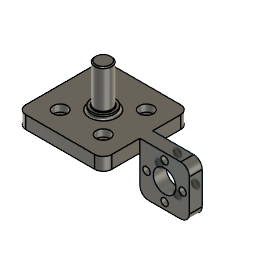
MGN12H_Carriage_Adapter (Autodesk Fusion 360 design; units mm, degrees)
part number: 2026-08-12-12-25-13-013
Autodesk Fusion 360 part; units mm, degrees
sketch "草图1" plane through (0, 0, 0) normal (0, 0, 1) x (1, 0, 0)
  line L0 (20, 20) -> (-20, 20)
  line L1 (-20, 20) -> (-20, -20)
  line L2 (-20, -20) -> (20, -20)
  line L3 (20, -20) -> (20, 20)
  line L4 (20, 20) -> (-20, -20) construction
  line L5 (-20, 20) -> (20, -20) construction
  dimension "d25" = 40
  dimension "d26" = 40
  constraint horizontal L0
  constraint perpendicular L0 L1
  constraint parallel L0 L2
  constraint parallel L1 L3
  constraint coincident L4 origin
  constraint coincident L5 origin
  measures "d25" distance of L0.start L0.end
  measures "d26" distance of L0.start L2.end
extrude "拉伸1" add sketch "草图1" along normal blind 6
fillet "圆角1" radius 4 4 edges at (-20, -20, 3) (20, -20, 3) (20, 20, 3) (-20, 20, 3)
sketch "草图2" plane through (0, 0, 6) normal (0, 0, 1) x (-1, 0, 0)
  arc A0 (16, -20) -> (20, -16) centre (16, -16) ccw
  line L0 (20, -16) -> (20, 16)
  arc A1 (20, 16) -> (16, 20) centre (16, 16) ccw
  line L1 (16, 20) -> (-16, 20)
  arc A2 (-16, 20) -> (-20, 16) centre (-16, 16) ccw
  line L2 (-20, 16) -> (-20, -16)
  arc A3 (-20, -16) -> (-16, -20) centre (-16, -16) ccw
  line L3 (-16, -20) -> (16, -20)
  point P0 (-10, -10)
  dimension "d31" = 10
  dimension "d32" = 10
  measures "d31" distance of L2 P0
  measures "d32" distance of L3 P0
hole "孔1" at (10, 10, 6) direction (0, 0, -1) diameter 3.4 depth 15 tip angle 118 counterbore diameter 6.5 counterbore depth 3.3
pattern_linear "R-阵列1" count 2 spacing 20 along (-1, 0, 0) count 2 spacing 20 along (0, -1, 0) of "孔1"
sketch "草图3" plane through (0, 0, 6) normal (0, 0, 1) x (-1, 0, 0)
  circle A0 centre (10, 10) radius 3.25
  circle A1 centre (-10, 10) radius 3.25
  circle A2 centre (10, -10) radius 3.25
  circle A3 centre (-10, -10) radius 3.25
  arc A4 (16, -20) -> (20, -16) centre (16, -16) ccw
  line L0 (20, -16) -> (20, 16)
  arc A5 (20, 16) -> (16, 20) centre (16, 16) ccw
  line L1 (16, 20) -> (-16, 20)
  arc A6 (-16, 20) -> (-20, 16) centre (-16, 16) ccw
  line L2 (-20, 16) -> (-20, -16)
  arc A7 (-20, -16) -> (-16, -20) centre (-16, -16) ccw
  line L3 (-16, -20) -> (16, -20)
  circle A8 centre (0, 0) radius 5.4
  dimension "d42" = 10.8
  constraint coincident A8.centre origin
  measures "d42" diameter of A8
extrude "拉伸2" add sketch "草图3" along normal blind 1.8 contours A8
fillet "圆角2" radius 1 1 edges at (5.0346, -1.9527, 6)
sketch "草图4" plane through (0, 0, 7.8) normal (0, 0, 1) x (-1, 0, 0)
  circle A0 centre (0, 0) radius 5.4
  circle A1 centre (0, 0) radius 3.95
  dimension "d47" = 7.9
  constraint coincident A0.centre A1.centre
  measures "d47" diameter of A1
extrude "拉伸3" add sketch "草图4" along normal blind 18 contours A1
fillet "圆角3" radius 0.3 1 edges at (3.6827, -1.4284, 7.8)
chamfer "倒角1" distance 0.5 angle 45 1 edges at (3.6827, 1.4284, 25.8)
sketch "草图5" plane through (0, 0, 0) normal (0, 1, 0) x (1, 0, 0)
sketch "草图6" plane through (0, 0, 0) normal (0, 0, 1) x (1, 0, 0)
  line L0 (20, -3) -> (43, -3)
  line L1 (43, -3) -> (43, 3)
  line L2 (43, 3) -> (20, 3)
  line L3 (20, 3) -> (20, -3)
  constraint horizontal L0
  constraint vertical L1
  constraint horizontal L2
  constraint vertical L3
extrude "拉伸4" add sketch "草图6" along normal blind 6 and the other way blind 17
sketch "草图7" plane through (0, 3, 0) normal (0, 1, 0) x (-1, 0, 0)
  line L0 (-20, 0) -> (-20, 6)
  line L1 (-20, 6) -> (-43, 6)
  line L2 (-43, 6) -> (-43, -17)
  line L3 (-43, -17) -> (-20, -17)
  line L4 (-20, -17) -> (-20, 0)
  circle A0 centre (-31.5, -5.5) radius 5.25
  line L5 (0, 20) -> (0, 2.5)
  dimension "d57" = 10.5
  dimension "d58" = 31.5
  dimension "d59" = 11.5
  measures "d57" diameter of A0
  measures "d58" distance of A0.centre L5
  measures "d59" distance of L1 A0.centre
extrude "拉伸5" cut sketch "草图7" against normal blind 6 contours A0
sketch "草图8" plane through (0, 3, 0) normal (0, 1, 0) x (-1, 0, 0)
  circle A0 centre (-31.5, -5.5) radius 5.25
  line L0 (-20, 0) -> (-20, 6)
  line L1 (-20, 6) -> (-43, 6)
  line L2 (-43, 6) -> (-43, -17)
  line L3 (-43, -17) -> (-20, -17)
  line L4 (-20, -17) -> (-20, 0)
  circle A1 centre (-31.5, 2.875) radius 1.7
  circle A2 centre (-31.5, -13.875) radius 1.7
  circle A3 centre (-39.875, -5.5) radius 1.7
  circle A4 centre (-23.125, -5.5) radius 1.7
  dimension "d62" = 3.4
  dimension "d64" = 3.125
  dimension "d67" = 11.5
  dimension "d68" = 3.4
  dimension "d69" = 3.125
  dimension "d70" = 11.5
  dimension "d71" = 3.4
  dimension "d72" = 3.4
  dimension "d73" = 3.125
  dimension "d74" = 3.125
  dimension "d75" = 11.5
  dimension "d76" = 11.5
  measures "d62" diameter of A1
  measures "d64" distance of L1 A1.centre
  measures "d67" distance of L0 A1.centre
  measures "d68" diameter of A2
  measures "d69" distance of L3 A2.centre
  measures "d70" distance of L4 A2.centre
  measures "d71" diameter of A3
  measures "d72" diameter of A4
  measures "d73" distance of L2 A3.centre
  measures "d74" distance of L4 A4.centre
  measures "d75" distance of L3 A3.centre
  measures "d76" distance of L3 A4.centre
extrude "拉伸7" cut sketch "草图8" against normal blind 6 contours A1 | A2 | A3 | A4
fillet "圆角4" radius 4 3 edges at (43, 0, 6) (43, 0, -17) (20, 0, -17)
equation "Base_Length = 40 mm" comment "Base length"
equation "Base_Width = 40 mm" comment "Base width"
equation "Base_Thickness = 6 mm" comment "Base thickness"
equation "Base_Corner_Radius = 4 mm" comment "Base corner radius"
equation "Hole_Pitch_X = 20 mm" comment "M3 hole pitch X"
equation "Hole_Pitch_Y = 20 mm" comment "M3 hole pitch Y"
equation "M3_Clearance_Diameter = 3.4 mm" comment "M3 clearance hole diameter"
equation "Counterbore_Diameter = 6.5 mm" comment "M3 socket-head counterbore diameter"
equation "Counterbore_Depth = 3.3 mm" comment "M3 counterbore depth"
equation "Shaft_Diameter = 7.9 mm" comment "Vertical printed shaft diameter"
equation "Shoulder_Diameter = 10.8 mm" comment "Bearing inner-ring support shoulder diameter"
equation "Shoulder_Height = 1.8 mm" comment "Bearing shoulder height"
equation "Shaft_Height = 18 mm" comment "Shaft height above shoulder"
equation "Shoulder_Base_Fillet = 1 mm" comment "Fillet between shoulder and base"
equation "Shaft_Shoulder_Fillet = 0.3 mm" comment "Small fillet between shaft and shoulder"
equation "Shaft_Top_Chamfer = 0.5 mm" comment "Shaft top lead-in chamfer"
equation "Bearing_Width = 7 mm" comment "608 bearing width"
equation "Bearing_Stack_Width = Bearing_Width * 2" comment "Two 608 bearings total width"
equation "Top_Retention_Hole_Diameter = 2.2 mm" comment "Transverse retention hole diameter"
equation "Top_Retention_Hole_Height = 15.5 mm" comment "Hole center height above shoulder"
equation "Axial_Clearance_Target = 0.6 mm" comment "Target axial play under retention pin"
equation "Bearing_ID = 8 mm" comment "608 bearing nominal inner diameter"
equation "Bearing_OD = 22 mm" comment "608 bearing nominal outer diameter"
equation "Wheel_Base_Clearance_Target = 1.5 mm" comment "Target wheel-to-base clearance"
equation "d25 = Base_Length"
equation "d26 = Base_Width"
equation "d27 = Base_Thickness"
equation "d30 = Base_Corner_Radius"
equation "d31 = ( Base_Length - Hole_Pitch_X ) / 2"
equation "d32 = ( Base_Width - Hole_Pitch_Y ) / 2"
equation "d34 = M3_Clearance_Diameter"
equation "d36 = Counterbore_Depth"
equation "d37 = Counterbore_Diameter"
equation "d40 = Hole_Pitch_X"
equation "d41 = Hole_Pitch_Y"
equation "d42 = Shoulder_Diameter"
equation "d43 = Shoulder_Height"
equation "d46 = Shoulder_Base_Fillet"
equation "d47 = Shaft_Diameter"
equation "d48 = Shaft_Height"
equation "d51 = Shaft_Shoulder_Fillet"
equation "d52 = Shaft_Top_Chamfer"
equation "d58 = ( 23 / 2 ) * 1 mm + 20 mm"
equation "d59 = ( 23 / 2 ) * 1 mm"
equation "d64 = ( ( 23 / 2 - 10.5 / 2 ) / 2 ) * 1 mm"
equation "d67 = ( 23 / 2 ) * 1 mm"
equation "d80 = Base_Corner_Radius"
